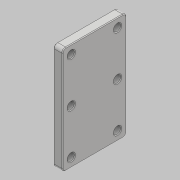
# Autodesk Inventor part: exercise3-16ipt
Saved by Autodesk Inventor 2018 (Build 220112000, 112)
## iProperties
Created: 2020-09-23
Part Number: exercise3-16ipt
Material: 一般
Document SubType Name: Modeling
Designer: 王鼎鈞
Density: 1 g/cm^3
Appearance: 預設
Author: 王鼎鈞
Autodesk Inventor part; units mm, degrees
ref_plane "YZ Plane" through (0, 0, 0) normal (1, 0, 0) x (0, 1, 0)
ref_plane "XZ Plane" through (0, 0, 0) normal (0, 1, 0) x (-1, 0, 0)
sketch "草圖1" plane through (0, 0, 0) normal (1, 0, 0) x (0, 1, 0)
  line L0 (-90, 150) -> (90, 150)
  line L1 (90, 150) -> (90, -150)
  line L2 (90, -150) -> (-90, -150)
  line L3 (-90, -150) -> (-90, 150)
  line L4 (-90, 150) -> (90, -150) construction
  line L5 (90, 150) -> (-90, -150) construction
  point P0 (0, 0)
  dimension "d0" = 180
  dimension "d1" = 300
  constraints: 12 end point, 2 midpoint, 2 parallel, 1 horizontal, 1 perpendicular
  measures "d0" distance of L1.end L2.end
  measures "d1" distance of L0.end L1.end
extrude "擠出1" add sketch "草圖1" along normal blind 25
fillet "圓角1" radius 10 4 edges at (12.5, 90, 150) (12.5, -90, 150) (12.5, 90, -150) (12.5, -90, -150)
chamfer "倒角1" distance 2 angle 45 16 edges at (25, 90, 0) (25, 87.0711, 147.0711) (25, 0, 150) (25, -87.0711, 147.0711) (25, -90, 0) (25, -87.0711, -147.0711) (25, 0, -150) (25, 87.0711, -147.0711) (0, 90, 0) (0, 87.0711, -147.0711) (0, 0, -150) (0, -87.0711, -147.0711) (0, -90, 0) (0, -87.0711, 147.0711) (0, 0, 150) (0, 87.0711, 147.0711)
sketch "草圖2" plane through (25, 0, 0) normal (1, 0, 0) x (0, 0, -1)
  line L0 (-150, 80) -> (-150, -80) projected
  line L1 (0, -126) -> (0, 126) projected
  line L2 (210, 0) -> (-210, 0) projected
  line L3 (-125, -126) -> (-125, 126)
  line L4 (210, 65) -> (-210, 65)
  point P0 (0, 0)
  point P1 (-125, 65)
  dimension "d8" = 125
  dimension "d9" = 65
  constraints: 4 end point, 2 parallel, 2 point on line
  measures "d8" distance between parallel lines of L1 L3
  measures "d9" distance between parallel lines of L2 L4
hole "孔1" at (25, 65, 125) direction (-1, 0, 0) diameter 20 end through all
chamfer "倒角2" distance 2 angle 45 2 edges at (25, 65, 135) (0, 65, 135)
pattern_linear "矩形陣列1" count 3 spacing 125 along (0, 0, -1) of "孔1", "倒角2"
ref_plane "工作平面1" through (2, 0, -140) normal (0, -1, 0) x (1, 0, 0)
mirror "鏡射1" about plane through (2, 0, -140) normal (0, -1, 0) of "孔1", "倒角2", "矩形陣列1"
